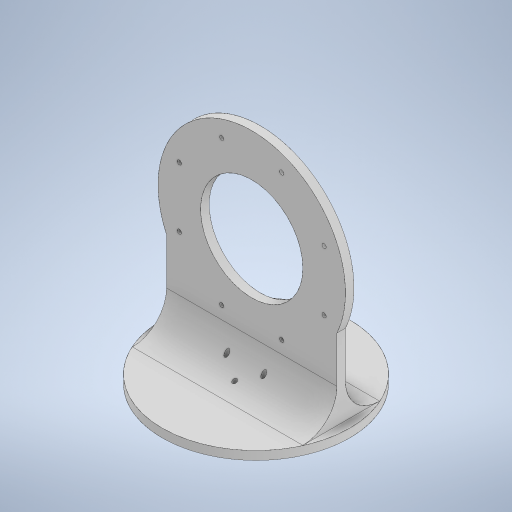
# Autodesk Inventor part: legparts_07(five)
Saved by Autodesk Inventor 2024.3 (Build 283343000, 343)
## iProperties
Created: 2024-10-21
Part Number: legparts_07(five)
Material: 一般
Document SubType Name: Modeling
Designer: 佐藤智貴
Density: 1 g/cm^3
Appearance: 既定
Mass: 104.488 g
Surface Area: 473.803 cm^2
Volume: 104.488 cm^3
Author: 佐藤智貴
Autodesk Inventor part; units mm, degrees
ref_plane "YZ Plane" through (0, 0, 0) normal (1, 0, 0) x (0, 1, 0)
ref_plane "XZ Plane" through (0, 0, 0) normal (0, 1, 0) x (-1, 0, 0)
ref_plane "XY Plane" through (0, 0, 0) normal (0, 0, 1) x (1, 0, 0)
sketch "スケッチ1" plane through (0, 0, 0) normal (0, 0, 1) x (1, 0, 0)
  circle A0 centre (0, 0) radius 48.5
  circle A1 centre (0, 0) radius 30
  line L0 (-50, 50) -> (50, 50)
  line L1 (50, 50) -> (50, -50)
  line L2 (50, -50) -> (-50, -50)
  line L3 (-50, -50) -> (-50, 50)
  line L4 (-50, -50) -> (50, -50)
  line L5 (50, -50) -> (50, -70)
  line L6 (50, -70) -> (-50, -70)
  line L7 (-50, -70) -> (-50, -50)
  circle A2 centre (0, 0) radius 55
  point P0 (-50, -60)
  point P1 (-50, -22.9129)
  point P2 (50, -22.9129)
  dimension "d0" = 97
  dimension "d3" = 50
  dimension "d4" = 50
  dimension "d5" = 50
  dimension "d6" = 50
  dimension "d126" = 20
  dimension "d127" = 100
  dimension "d128" = 110
  dimension "d129" = 60
  constraints: 16 end point, 4 parallel, 3 centre point, 2 horizontal, 2 perpendicular, 1 coincident, 1 midpoint
  measures "d0" diameter of A0
  measures "d3" distance from line of L0 point (0, 0)
  measures "d4" distance from line of L2 point (0, 0)
  measures "d5" distance from line of L1 point (0, 0)
  measures "d6" distance from line of point (0, 0) L3
  measures "d126" distance between parallel lines of L2 L6
  measures "d127" distance from line of point (-50, -60) L5
  measures "d128" diameter of A2
  measures "d129" diameter of A1
extrude "押し出し1" add sketch "スケッチ1" along normal blind 5 contours A0 | A1 | A2 L0 | L0 A2 L1 L2 L3 | L3 A2 | A2 L2 L3 | A2 L1 | L2 A2 L5 L6 L7 | L2 A2 | L1 L2 A2
sketch "スケッチ2" plane through (0, 0, 5) normal (0, 0, 1) x (1, 0, 0)
  circle A0 centre (0, 0) radius 46
  line L0 (0, 0) -> (0, 64.6511)
  line L1 (0, 0) -> (-25.9524, 62.6547)
  line L2 (-50, -22.9129) -> (-50, -70) projected
  point P0 (-17.6034, 42.4985)
  point P1 (-42.4985, 17.6034)
  point P2 (-42.4985, -17.6034)
  point P3 (-17.6034, -42.4985)
  point P4 (17.6034, -42.4985)
  point P5 (42.4985, -17.6034)
  point P6 (42.4985, 17.6034)
  point P7 (17.6034, 42.4985)
  point P8 (-50, 50)
  point P9 (-50, -50)
  dimension "d7" = 92
  dimension "d8" = 22.5
  dimension "d11" = 360
  dimension "d76" = 50
  constraints: 4 end point, 1 coincident, 1 point on line, 1 vertical, 12 other
  measures "d8" angle of L0 L1
  measures "d76" distance from line of L2 point (0, 0)
hole "穴1" at (-17.6034, 42.4985, 5) at (-42.4985, 17.6034, 5) at (-42.4985, -17.6034, 5) at (-17.6034, -42.4985, 5) at (17.6034, -42.4985, 5) at (42.4985, -17.6034, 5) at (42.4985, 17.6034, 5) at (17.6034, 42.4985, 5) direction (0, 0, -1) diameter 2.459 end through all
sketch "スケッチ3" plane through (0, 0, 5) normal (0, 0, 1) x (1, 0, 0)
  circle A0 centre (0, 0) radius 30
  dimension "d20" = 60
  constraints: 1 centre point, 1 coincident
  measures "d20" diameter of A0
extrude "押し出し2" cut sketch "スケッチ3" against normal blind 5
sketch "スケッチ16" plane through (0, 0, 0) normal (0, 0, -1) x (-1, 0, 0)
  circle A0 centre (17.6034, 42.4985) radius 1.2295 projected
  circle A1 centre (0, 0) radius 46
  circle A2 centre (17.6034, 42.4985) radius 3
  circle A3 centre (-17.6034, 42.4985) radius 3
  circle A4 centre (-42.4985, 17.6034) radius 3
  circle A5 centre (-42.4985, -17.6034) radius 3
  circle A6 centre (-17.6034, -42.4985) radius 3
  circle A7 centre (17.6034, -42.4985) radius 3
  circle A8 centre (42.4985, -17.6034) radius 3
  circle A9 centre (42.4985, 17.6034) radius 3
  point P0 (18.7653, 42.0962)
  point P1 (16.4975, 43.0356)
  dimension "d113" = 6
  dimension "d116" = 360
  constraints: 8 centre point, 2 coincident, 20 other
  measures "d113" diameter of A2
extrude "押し出し12" cut sketch "スケッチ16" against normal blind 2 contours A0 A1 | A0 A1 A2 | A1 A0 | A0 A1 A2 | A3 A1 | A1 A3 | A9 A1 | A1 A9 | A4 A1 | A1 A4 | A8 A1 | A1 A8 | A5 A1 | A1 A5 | A7 A1 | A1 A7 | A6 A1 | A1 A6
sketch "スケッチ19" plane through (-50, -70, 0) normal (0, -1, 0) x (1, 0, 0)
  line L0 (0, 5) -> (100, 5) projected
  line L1 (0, 5) -> (100, 5)
  line L2 (100, 5) -> (100, -47.5)
  line L3 (100, -47.5) -> (0, -47.5)
  line L4 (0, -47.5) -> (0, 5)
  line L5 (0, -47.5) -> (100, -47.5)
  line L6 (100, -47.5) -> (100, 52.5)
  line L7 (100, 52.5) -> (0, 52.5)
  line L8 (0, 52.5) -> (0, -47.5)
  circle A0 centre (50, 2.5) radius 55
  point P0 (50, 0)
  dimension "d130" = 100
  dimension "d131" = 47.5
  dimension "d132" = 100
  dimension "d136" = 110
  dimension "d137" = 50
  dimension "d138" = 50
  constraints: 16 end point, 4 parallel, 2 horizontal, 2 perpendicular, 1 centre point, 1 point on line
  measures "d130" distance between parallel lines of L7 L3
  measures "d131" distance between parallel lines of L7 L0
  measures "d132" distance between parallel lines of L8 L6
  measures "d136" diameter of A0
  measures "d137" distance from line of L7 A0.centre
  measures "d138" distance from line of L4 A0.centre
extrude "押し出し14" add sketch "スケッチ19" along normal blind 5 contours L8 A0 L7 L6 L0 | L0 L2 A0 L3 L4 | L4 A0 L8 | L6 A0 L2 | L3 A0 | A0 L7
fillet "フィレット6" radius 20 2 edges at (0, -70, 5) (0, -70, 0)
sketch "スケッチ20" plane through (0, -75, 2.5) normal (0, -1, 0) x (1, 0, 0)
  circle A0 centre (0, 0) radius 12.5
  line L0 (-10.8253, -6.25) -> (0, 0)
  line L1 (0, 0) -> (-14.9018, 0)
  point P0 (0, -2.5)
  point P1 (0, -12.5)
  point P2 (10.8253, -6.25)
  point P3 (10.8253, 6.25)
  point P4 (0, 12.5)
  point P5 (-10.8253, 6.25)
  dimension "d139" = 25
  dimension "d140" = 30
  dimension "d143" = 360
  constraints: 4 end point, 1 horizontal, 10 other
  measures "d140" angle of L0 L1
hole "穴5" at (-10.8253, -75, -3.75) at (0, -75, -10) at (10.8253, -75, -3.75) at (10.8253, -75, 8.75) at (0, -75, 15) at (-10.8253, -75, 8.75) direction (0, 1, 0) diameter 2.459 end through all
equation "\"d4\" = d3"
equation "\"d5\" = d3"
equation "\"d6\" = d5"
